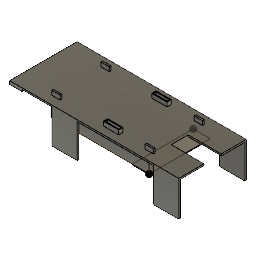
support v17 (Autodesk Fusion 360 design; units mm, degrees)
Autodesk Fusion 360 part; units mm, degrees
sketch "Sketch1" plane through (0, 0, 0) normal (0, 0, 1) x (1, 0, 0)
  line L0 (0, 0) -> (200, 0)
  line L1 (200, 0) -> (200, 80)
  line L2 (200, 80) -> (0, 80)
  line L3 (0, 80) -> (0, 0)
  dimension "d1" = 200
  dimension "d2" = 80
  dimension "d58" = 0
  dimension "d59" = 0
  dimension "d60" = 0
  dimension "d61" = 0
  dimension "d125" = 0
  dimension "d126" = 0
  dimension "d127" = 0
  dimension "d128" = 0
  constraint horizontal L0
  constraint vertical L1
  constraint horizontal L2
  constraint vertical L3
  constraint coincident L0.start L3.end
  measures "d1" distance of L0.start L0.end
  measures "d2" distance of L0.start L2.end
extrude "Extrude1" add sketch "Sketch1" along normal blind 2
sketch "Sketch2" plane through (0, 0, 2) normal (0, 0, 1) x (-1, 0, 0)
  line L0 (0, -80) -> (0, 0)
  line L1 (0, 0) -> (-200, 0)
  line L2 (-200, 0) -> (-200, -80)
  line L3 (-200, -80) -> (0, -80)
  line L4 (-40, -70) -> (-50, -70)
  line L5 (-50, -70) -> (-50, -68)
  line L6 (-50, -68) -> (-40, -68)
  line L7 (-40, -68) -> (-40, -70)
  dimension "d5" = 10
  dimension "d6" = 2
  dimension "d9" = 10
  dimension "d10" = 40
  constraint horizontal L4
  constraint vertical L5
  constraint horizontal L6
  constraint vertical L7
  measures "d5" distance of L4.start L4.end
  measures "d6" distance of L4.start L6.end
  measures "d9" distance of L3 L4
  measures "d10" distance of L0 L7
extrude "Extrude2" add sketch "Sketch2" along normal blind 5 contours L4 L5 L6 L7
sketch "Sketch3" plane through (0, 0, 2) normal (0, 0, 1) x (-1, 0, 0)
  line L0 (-40, -68) -> (-40, -70)
  line L1 (-40, -70) -> (-50, -70)
  line L2 (-50, -70) -> (-50, -68)
  line L3 (-50, -68) -> (-40, -68)
  line L4 (0, -80) -> (0, 0)
  line L5 (0, 0) -> (-200, 0)
  line L6 (-200, 0) -> (-200, -80)
  line L7 (-200, -80) -> (0, -80)
  line L8 (-40, -10) -> (-50, -10)
  line L9 (-50, -10) -> (-50, -12)
  line L10 (-50, -12) -> (-40, -12)
  line L11 (-40, -12) -> (-40, -10)
  dimension "d11" = 10
  dimension "d12" = 2
  dimension "d13" = 10
  dimension "d14" = 40
  constraint horizontal L8
  constraint vertical L9
  constraint horizontal L10
  constraint vertical L11
  measures "d11" distance of L8.start L8.end
  measures "d12" distance of L8.start L10.end
  measures "d13" distance of L5 L8
  measures "d14" distance of L4 L11
extrude "Extrude3" add sketch "Sketch3" along normal blind 5 contours L8 L9 L10 L11
sketch "Sketch4" plane through (0, 0, 2) normal (0, 0, 1) x (-1, 0, 0)
  line L0 (-40, -12) -> (-50, -12)
  line L1 (-50, -12) -> (-50, -10)
  line L2 (-50, -10) -> (-40, -10)
  line L3 (-40, -10) -> (-40, -12)
  line L4 (-40, -68) -> (-40, -70)
  line L5 (-40, -70) -> (-50, -70)
  line L6 (-50, -70) -> (-50, -68)
  line L7 (-50, -68) -> (-40, -68)
  line L8 (0, -80) -> (0, 0)
  line L9 (0, 0) -> (-200, 0)
  line L10 (-200, 0) -> (-200, -80)
  line L11 (-200, -80) -> (0, -80)
  line L12 (-160, -10) -> (-150, -10)
  line L13 (-150, -10) -> (-150, -12)
  line L14 (-150, -12) -> (-160, -12)
  line L15 (-160, -12) -> (-160, -10)
  dimension "d17" = 10
  dimension "d18" = 2
  dimension "d19" = 40
  dimension "d20" = 10
  constraint horizontal L12
  constraint vertical L13
  constraint horizontal L14
  constraint vertical L15
  measures "d17" distance of L12.start L12.end
  measures "d18" distance of L12.start L14.end
  measures "d19" distance of L10 L14.end
  measures "d20" distance of L9 L12
extrude "Extrude4" add sketch "Sketch4" along normal blind 5 contours L12 L13 L14 L15
sketch "Sketch5" plane through (0, 0, 2) normal (0, 0, 1) x (-1, 0, 0)
  line L0 (-160, -12) -> (-160, -10)
  line L1 (-160, -10) -> (-150, -10)
  line L2 (-150, -10) -> (-150, -12)
  line L3 (-150, -12) -> (-160, -12)
  line L4 (-40, -12) -> (-50, -12)
  line L5 (-50, -12) -> (-50, -10)
  line L6 (-50, -10) -> (-40, -10)
  line L7 (-40, -10) -> (-40, -12)
  line L8 (-40, -68) -> (-40, -70)
  line L9 (-40, -70) -> (-50, -70)
  line L10 (-50, -70) -> (-50, -68)
  line L11 (-50, -68) -> (-40, -68)
  line L12 (0, -80) -> (0, 0)
  line L13 (0, 0) -> (-200, 0)
  line L14 (-200, 0) -> (-200, -80)
  line L15 (-200, -80) -> (0, -80)
  line L16 (-160, -70) -> (-150, -70)
  line L17 (-150, -70) -> (-150, -68)
  line L18 (-150, -68) -> (-160, -68)
  line L19 (-160, -68) -> (-160, -70)
  dimension "d23" = 10
  dimension "d24" = 2
  dimension "d25" = 40
  dimension "d26" = 10
  constraint horizontal L16
  constraint vertical L17
  constraint horizontal L18
  constraint vertical L19
  measures "d23" distance of L16.start L16.end
  measures "d24" distance of L16.start L18.end
  measures "d25" distance of L14 L19
  measures "d26" distance of L15 L16
extrude "Extrude5" add sketch "Sketch5" along normal blind 5 contours L16 L17 L18 L19
sketch "Sketch8" plane through (0, 0, 0) normal (0, 0, 1) x (1, 0, 0)
  line L0 (45, 4) -> (160, 4)
  line L1 (160, 4) -> (160, 5)
  line L2 (160, 5) -> (45, 5)
  line L3 (45, 5) -> (45, 4)
  line L4 (0, 0) -> (200, 0)
  line L5 (0, 80) -> (0, 0)
  dimension "d42" = 115
  dimension "d43" = 1
  dimension "d44" = 4
  dimension "d45" = 45
  constraint horizontal L0
  constraint vertical L1
  constraint horizontal L2
  constraint vertical L3
  measures "d42" distance of L0.start L0.end
  measures "d43" distance of L0.start L2.end
  measures "d44" distance of L0 L4
  measures "d45" distance of L3 L5
extrude "Extrude8" add sketch "Sketch8" against normal blind 15
sketch "Sketch9" plane through (0, 0, 0) normal (0, 0, -1) x (1, 0, 0)
  line L0 (45, -4) -> (160, -4)
  line L1 (160, -4) -> (160, -5)
  line L2 (160, -5) -> (45, -5)
  line L3 (45, -5) -> (45, -4)
  line L4 (0, 0) -> (0, -80)
  line L5 (0, -80) -> (200, -80)
  line L6 (200, -80) -> (200, 0)
  line L7 (200, 0) -> (0, 0)
  line L8 (45, -76) -> (160, -76)
  line L9 (160, -76) -> (160, -75)
  line L10 (160, -75) -> (45, -75)
  line L11 (45, -75) -> (45, -76)
  dimension "d48" = 115
  dimension "d49" = 1
  dimension "d50" = 4
  dimension "d51" = 45
  constraint horizontal L8
  constraint vertical L9
  constraint horizontal L10
  constraint vertical L11
  measures "d48" distance of L8.start L8.end
  measures "d49" distance of L8.start L10.end
  measures "d50" distance of L5 L8
  measures "d51" distance of L4 L11
extrude "Extrude9" add sketch "Sketch9" along normal blind 15 contours L8 L9 L10 L11
sketch "Sketch10" plane through (0, 0, 0) normal (0, 0, -1) x (1, 0, 0)
  line L0 (45, -75) -> (160, -75)
  line L1 (160, -75) -> (160, -76)
  line L2 (160, -76) -> (45, -76)
  line L3 (45, -76) -> (45, -75)
  line L4 (45, -4) -> (160, -4)
  line L5 (160, -4) -> (160, -5)
  line L6 (160, -5) -> (45, -5)
  line L7 (45, -5) -> (45, -4)
  line L8 (0, 0) -> (0, -80)
  line L9 (0, -80) -> (200, -80)
  line L10 (200, -80) -> (200, 0)
  line L11 (200, 0) -> (0, 0)
  line L12 (200, -80) -> (170, -80)
  line L13 (170, -80) -> (170, -78)
  line L14 (170, -78) -> (200, -78)
  line L15 (200, -78) -> (200, -80)
  dimension "d66" = 30
  dimension "d67" = 2
  constraint horizontal L12
  constraint vertical L13
  constraint horizontal L14
  constraint vertical L15
  constraint coincident L9.end L10.start
  measures "d66" distance of L9.end L12.end
  measures "d67" distance of L9.end L14.end
extrude "Extrude10" add sketch "Sketch10" along normal blind 40 contours L9 L10 L12 L13 L14 L15
sketch "Sketch11" plane through (0, 0, 0) normal (0, 0, -1) x (1, 0, 0)
  line L0 (170, -80) -> (170, -78)
  line L1 (170, -78) -> (200, -78)
  line L2 (200, -78) -> (200, 0)
  line L3 (200, 0) -> (0, 0)
  line L4 (0, 0) -> (0, -80)
  line L5 (0, -80) -> (170, -80)
  line L6 (45, -4) -> (160, -4)
  line L7 (160, -4) -> (160, -5)
  line L8 (160, -5) -> (45, -5)
  line L9 (45, -5) -> (45, -4)
  line L10 (45, -75) -> (160, -75)
  line L11 (160, -75) -> (160, -76)
  line L12 (160, -76) -> (45, -76)
  line L13 (45, -76) -> (45, -75)
  line L14 (200, 0) -> (170, 0)
  line L15 (170, 0) -> (170, -2)
  line L16 (170, -2) -> (200, -2)
  line L17 (200, -2) -> (200, 0)
  dimension "d70" = 2
  dimension "d71" = 30
  constraint horizontal L14
  constraint vertical L15
  constraint horizontal L16
  constraint vertical L17
  constraint coincident L2.end L3.start
  measures "d70" distance of L2.end L16.end
  measures "d71" distance of L2.end L14.end
extrude "Extrude11" add sketch "Sketch11" along normal blind 40 contours L2 L3 L14 L15 L16 L17
sketch "Sketch12" plane through (0, 0, 0) normal (0, 0, -1) x (1, 0, 0)
  line L0 (170, -2) -> (170, 0)
  line L1 (170, 0) -> (0, 0)
  line L2 (0, 0) -> (0, -80)
  line L3 (0, -80) -> (170, -80)
  line L4 (170, -80) -> (170, -78)
  line L5 (170, -78) -> (200, -78)
  line L6 (200, -78) -> (200, -2)
  line L7 (200, -2) -> (170, -2)
  line L8 (45, -4) -> (160, -4)
  line L9 (160, -4) -> (160, -5)
  line L10 (160, -5) -> (45, -5)
  line L11 (45, -5) -> (45, -4)
  line L12 (45, -75) -> (160, -75)
  line L13 (160, -75) -> (160, -76)
  line L14 (160, -76) -> (45, -76)
  line L15 (45, -76) -> (45, -75)
  line L16 (50, 0) -> (80, 0)
  line L17 (80, 0) -> (80, -2)
  line L18 (80, -2) -> (50, -2)
  line L19 (50, -2) -> (50, 0)
  dimension "d74" = 30
  dimension "d75" = 2
  dimension "d78" = 50
  constraint horizontal L16
  constraint vertical L17
  constraint horizontal L18
  constraint vertical L19
  constraint coincident L1 L16.start
  measures "d74" distance of L16.start L16.end
  measures "d75" distance of L16.start L18.end
  measures "d78" distance of L2 L19
extrude "Extrude12" add sketch "Sketch12" along normal blind 40 contours L1 L16 L17 L18 L19
sketch "Sketch13" plane through (0, 0, 0) normal (0, 0, -1) x (1, 0, 0)
  line L0 (45, -75) -> (160, -75)
  line L1 (160, -75) -> (160, -76)
  line L2 (160, -76) -> (45, -76)
  line L3 (45, -76) -> (45, -75)
  line L4 (45, -4) -> (160, -4)
  line L5 (160, -4) -> (160, -5)
  line L6 (160, -5) -> (45, -5)
  line L7 (45, -5) -> (45, -4)
  line L8 (80, 0) -> (80, -2)
  line L9 (80, -2) -> (50, -2)
  line L10 (50, -2) -> (50, 0)
  line L11 (50, 0) -> (0, 0)
  line L12 (0, 0) -> (0, -80)
  line L13 (0, -80) -> (170, -80)
  line L14 (170, -80) -> (170, -78)
  line L15 (170, -78) -> (200, -78)
  line L16 (200, -78) -> (200, -2)
  line L17 (200, -2) -> (170, -2)
  line L18 (170, -2) -> (170, 0)
  line L19 (170, 0) -> (80, 0)
  line L20 (50, -80) -> (80, -80)
  line L21 (80, -80) -> (80, -78)
  line L22 (80, -78) -> (50, -78)
  line L23 (50, -78) -> (50, -80)
  point P0 (200, -78)
  point P1 (200, -2)
  dimension "d79" = 30
  dimension "d80" = 2
  dimension "d81" = 50
  dimension "d175" = 76
  constraint horizontal L20
  constraint vertical L21
  constraint horizontal L22
  constraint vertical L23
  constraint coincident L13 L20.start
  measures "d79" distance of L20.start L20.end
  measures "d80" distance of L20.start L22.end
  measures "d81" distance of L12 L23
  measures "d175" distance of P0 P1
extrude "Extrude13" add sketch "Sketch13" along normal blind 40 contours L13 L20 L21 L22 L23
sketch "Sketch17" plane through (200, 0, 0) normal (1, 0, 0) x (0, 1, 0)
  line L0 (2, 0) -> (78, 0)
  line L1 (78, 0) -> (78, -40)
  line L2 (78, -40) -> (80, -40)
  line L3 (80, -40) -> (80, 2)
  line L4 (80, 2) -> (0, 2)
  line L5 (0, 2) -> (0, -40)
  line L6 (0, -40) -> (2, -40)
  line L7 (2, -40) -> (2, 0)
  line L8 (30, 2) -> (50, 2)
  line L9 (50, 2) -> (50, 0)
  line L10 (50, 0) -> (30, 0)
  line L11 (30, 0) -> (30, 2)
  dimension "d115" = 20
  dimension "d116" = 2
  dimension "d117" = 30
  dimension "d118" = 28.4712
  constraint horizontal L8
  constraint vertical L9
  constraint horizontal L10
  constraint vertical L11
  constraint coincident L4 L8.start
  measures "d115" distance of L8.start L8.end
  measures "d116" distance of L8.start L10.end
  measures "d117" distance of L5 L8.start
extrude "Extrude15" cut sketch "Sketch17" against normal blind 39 contours L0 L4 L8 L9 L10 L11
sketch "Sketch21" plane through (0, 0, 0) normal (0, 0, -1) x (1, 0, 0)
  line L0 (45, -4) -> (160, -4)
  line L1 (160, -4) -> (160, -5)
  line L2 (160, -5) -> (45, -5)
  line L3 (45, -5) -> (45, -4)
  line L4 (45, -75) -> (160, -75)
  line L5 (160, -75) -> (160, -76)
  line L6 (160, -76) -> (45, -76)
  line L7 (45, -76) -> (45, -75)
  line L8 (200, -50) -> (161, -50)
  line L9 (161, -50) -> (161, -30)
  line L10 (161, -30) -> (200, -30)
  line L11 (200, -30) -> (200, -2)
  line L12 (200, -2) -> (170, -2)
  line L13 (170, -2) -> (170, 0)
  line L14 (170, 0) -> (80, 0)
  line L15 (80, 0) -> (80, -2)
  line L16 (80, -2) -> (50, -2)
  line L17 (50, -2) -> (50, 0)
  line L18 (50, 0) -> (0, 0)
  line L19 (0, 0) -> (0, -80)
  line L20 (0, -80) -> (50, -80)
  line L21 (50, -80) -> (50, -78)
  line L22 (50, -78) -> (80, -78)
  line L23 (80, -78) -> (80, -80)
  line L24 (80, -80) -> (170, -80)
  line L25 (170, -80) -> (170, -78)
  line L26 (170, -78) -> (200, -78)
  line L27 (200, -78) -> (200, -50)
  line L28 (0, -80) -> (15, -80)
  line L29 (15, -80) -> (15, 0)
  line L30 (15, 0) -> (0, 0)
  line L31 (0, 0) -> (0, -80)
  constraint horizontal L28
  constraint vertical L29
  constraint horizontal L30
  constraint vertical L31
  constraint coincident L18 L29.end
  constraint coincident L19.end L20.start
extrude "Extrude20" add sketch "Sketch21" along normal blind 2 contours L18 L19 L20 L28 L29 L30 L31
sketch "Sketch23" plane through (0, 0, -2) normal (0, 0, -1) x (1, 0, 0)
  line L0 (0, 0) -> (0, -80)
  line L1 (0, -80) -> (15, -80)
  line L2 (15, -80) -> (15, 0)
  line L3 (15, 0) -> (0, 0)
  line L4 (15, -40) -> (0, -40)
  line L5 (0, -40) -> (0, -48)
  line L6 (0, -48) -> (15, -48)
  line L7 (15, -48) -> (15, -40)
  dimension "d168" = 8
  constraint horizontal L4
  constraint vertical L5
  constraint horizontal L6
  constraint vertical L7
  constraint midpoint L2 L4.start
  measures "d168" distance of L4.start L6.end
extrude "Extrude21" add sketch "Sketch23" along normal blind 1 contours L0 L2 L4 L5 L6 L7
sketch "Sketch26" plane through (0, 0, 0) normal (0, 0, -1) x (1, 0, 0)
  line L0 (15, 0) -> (15, -80)
  line L1 (15, -80) -> (50, -80)
  line L2 (50, -80) -> (50, -78)
  line L3 (50, -78) -> (80, -78)
  line L4 (80, -78) -> (80, -80)
  line L5 (80, -80) -> (170, -80)
  line L6 (170, -80) -> (170, -78)
  line L7 (170, -78) -> (200, -78)
  line L8 (200, -78) -> (200, -50)
  line L9 (200, -50) -> (161, -50)
  line L10 (161, -50) -> (161, -30)
  line L11 (161, -30) -> (200, -30)
  line L12 (200, -30) -> (200, -2)
  line L13 (200, -2) -> (170, -2)
  line L14 (170, -2) -> (170, 0)
  line L15 (170, 0) -> (80, 0)
  line L16 (80, 0) -> (80, -2)
  line L17 (80, -2) -> (50, -2)
  line L18 (50, -2) -> (50, 0)
  line L19 (50, 0) -> (15, 0)
  line L20 (45, -4) -> (160, -4)
  line L21 (160, -4) -> (160, -5)
  line L22 (160, -5) -> (45, -5)
  line L23 (45, -5) -> (45, -4)
  line L24 (45, -75) -> (160, -75)
  line L25 (160, -75) -> (160, -76)
  line L26 (160, -76) -> (45, -76)
  line L27 (45, -76) -> (45, -75)
  line L28 (160, -76) -> (161, -76)
  line L29 (161, -76) -> (161, -4)
  line L30 (161, -4) -> (160, -4)
  line L31 (160, -4) -> (160, -76)
  dimension "d178" = 1
  constraint horizontal L28
  constraint vertical L29
  constraint horizontal L30
  constraint vertical L31
  constraint coincident L25.end L26.start
  measures "d178" distance of L25.end L28.end
extrude "Extrude22" add sketch "Sketch26" along normal blind 15 contours L10 L21 L25 L28 L29 L30 L31
sketch "Sketch28" plane through (0, 0, -15) normal (0, 0, -1) x (1, 0, 0)
  line L0 (45, -75) -> (45, -76)
  line L1 (45, -76) -> (161, -76)
  line L2 (161, -76) -> (161, -4)
  line L3 (161, -4) -> (45, -4)
  line L4 (45, -4) -> (45, -5)
  line L5 (45, -5) -> (160, -5)
  line L6 (160, -5) -> (160, -75)
  line L7 (160, -75) -> (45, -75)
  line L8 (161, -4) -> (141, -4)
  line L9 (141, -4) -> (141, -76)
  line L10 (141, -76) -> (161, -76)
  line L11 (161, -76) -> (161, -4)
  dimension "d185" = 20
  constraint horizontal L8
  constraint vertical L9
  constraint horizontal L10
  constraint vertical L11
  constraint coincident L1 L9.end
  constraint coincident L2.end L3.start
  measures "d185" distance of L9 L11
extrude "Extrude25" add sketch "Sketch28" along normal blind 1 contours L5 L6 L7 L9 | L1 L2 L3 L5 L6 L7 L8 L9 L10 L11
sketch "Sketch29" plane through (0, 0, 2) normal (0, 0, 1) x (-1, 0, 0)
  line L0 (-161, -50) -> (-200, -50)
  line L1 (-200, -50) -> (-200, -80)
  line L2 (-200, -80) -> (0, -80)
  line L3 (0, -80) -> (0, 0)
  line L4 (0, 0) -> (-200, 0)
  line L5 (-200, 0) -> (-200, -30)
  line L6 (-200, -30) -> (-161, -30)
  line L7 (-161, -30) -> (-161, -50)
  line L8 (-160, -68) -> (-150, -68)
  line L9 (-150, -68) -> (-150, -70)
  line L10 (-150, -70) -> (-160, -70)
  line L11 (-160, -70) -> (-160, -68)
  line L12 (-160, -12) -> (-160, -10)
  line L13 (-160, -10) -> (-150, -10)
  line L14 (-150, -10) -> (-150, -12)
  line L15 (-150, -12) -> (-160, -12)
  line L16 (-40, -12) -> (-50, -12)
  line L17 (-50, -12) -> (-50, -10)
  line L18 (-50, -10) -> (-40, -10)
  line L19 (-40, -10) -> (-40, -12)
  line L20 (-40, -68) -> (-40, -70)
  line L21 (-40, -70) -> (-50, -70)
  line L22 (-50, -70) -> (-50, -68)
  line L23 (-50, -68) -> (-40, -68)
  line L24 (-120, -71) -> (-102, -71)
  line L25 (-102, -71) -> (-102, -66)
  line L26 (-102, -66) -> (-120, -66)
  line L27 (-120, -66) -> (-120, -71)
  line L28 (-103, -67) -> (-119, -67)
  line L29 (-119, -67) -> (-119, -70)
  line L30 (-119, -70) -> (-103, -70)
  line L31 (-103, -70) -> (-103, -67)
  dimension "d190" = 18
  dimension "d191" = 5
  dimension "d192" = 80
  dimension "d193" = 9
  dimension "d194" = 1
  dimension "d195" = 1
  constraint horizontal L24
  constraint vertical L25
  constraint horizontal L26
  constraint vertical L27
  constraint horizontal L28
  constraint vertical L29
  constraint horizontal L30
  constraint vertical L31
  measures "d190" distance of L24.start L24.end
  measures "d191" distance of L24.start L26.end
  measures "d192" distance of L1 L27
  measures "d193" distance of L2 L24
  measures "d194" distance of L24 L30
  measures "d195" distance of L25 L31
extrude "Extrude26" add sketch "Sketch29" along normal blind 5 contours L24 L25 L26 L27
sketch "Sketch30" plane through (0, 0, 2) normal (0, 0, 1) x (-1, 0, 0)
  line L0 (-40, -68) -> (-40, -70)
  line L1 (-40, -70) -> (-50, -70)
  line L2 (-50, -70) -> (-50, -68)
  line L3 (-50, -68) -> (-40, -68)
  line L4 (-40, -12) -> (-50, -12)
  line L5 (-50, -12) -> (-50, -10)
  line L6 (-50, -10) -> (-40, -10)
  line L7 (-40, -10) -> (-40, -12)
  line L8 (-160, -12) -> (-160, -10)
  line L9 (-160, -10) -> (-150, -10)
  line L10 (-150, -10) -> (-150, -12)
  line L11 (-150, -12) -> (-160, -12)
  line L12 (-160, -68) -> (-150, -68)
  line L13 (-150, -68) -> (-150, -70)
  line L14 (-150, -70) -> (-160, -70)
  line L15 (-160, -70) -> (-160, -68)
  line L16 (-161, -50) -> (-200, -50)
  line L17 (-200, -50) -> (-200, -80)
  line L18 (-200, -80) -> (0, -80)
  line L19 (0, -80) -> (0, 0)
  line L20 (0, 0) -> (-200, 0)
  line L21 (-200, 0) -> (-200, -30)
  line L22 (-200, -30) -> (-161, -30)
  line L23 (-161, -30) -> (-161, -50)
  line L24 (-120, -66) -> (-102, -66)
  line L25 (-102, -66) -> (-102, -71)
  line L26 (-102, -71) -> (-120, -71)
  line L27 (-120, -71) -> (-120, -66)
  line L28 (-120, -14) -> (-102, -14)
  line L29 (-102, -14) -> (-102, -9)
  line L30 (-102, -9) -> (-120, -9)
  line L31 (-120, -9) -> (-120, -14)
  line L32 (-103, -13) -> (-119, -13)
  line L33 (-119, -13) -> (-119, -10)
  line L34 (-119, -10) -> (-103, -10)
  line L35 (-103, -10) -> (-103, -13)
  dimension "d198" = 18
  dimension "d199" = 5
  dimension "d200" = 1
  dimension "d201" = 9
  constraint horizontal L28
  constraint vertical L29
  constraint horizontal L30
  constraint vertical L31
  constraint horizontal L32
  constraint vertical L33
  constraint horizontal L34
  constraint vertical L35
  measures "d198" distance of L28.start L28.end
  measures "d199" distance of L28.start L30.end
  measures "d200" distance of L28 L32
  measures "d201" distance of L20 L30
extrude "Extrude27" add sketch "Sketch30" along normal blind 5 contours L28 L29 L30 L31
